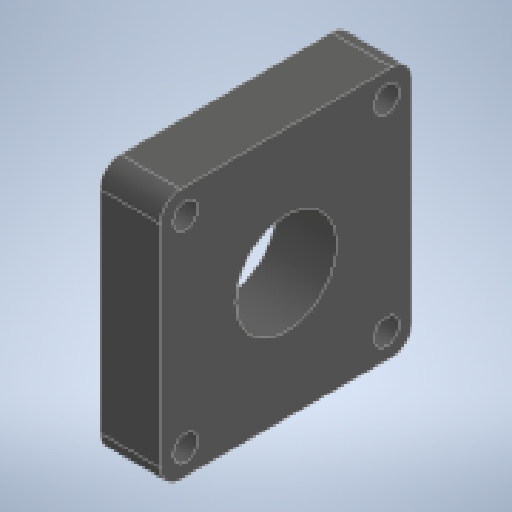
# Autodesk Inventor part: 25mmx25mmx6mm_fan
Saved by Autodesk Inventor 2024.1 (Build 281209000, 209)
## iProperties
Created: 2023-10-17
Part Number: 25mmx25mmx6mm_fan
Material: Generic
Document SubType Name: Modeling
Designer: l1534
Density: 1 g/cm^3
Appearance: Generic
Author: l1534
Autodesk Inventor part; units mm, degrees
ref_plane "YZ Plane" through (0, 0, 0) normal (1, 0, 0) x (0, 1, 0)
ref_plane "XZ Plane" through (0, 0, 0) normal (0, 1, 0) x (-1, 0, 0)
ref_plane "XY Plane" through (0, 0, 0) normal (0, 0, 1) x (1, 0, 0)
sketch "Sketch1" plane through (0, 0, 0) normal (1, 0, 0) x (0, 1, 0)
  line L0 (12.7439, 15.061) -> (-12.2561, 15.061)
  line L1 (-12.2561, 15.061) -> (-12.2561, -9.939)
  line L2 (-12.2561, -9.939) -> (12.7439, -9.939)
  line L3 (12.7439, -9.939) -> (12.7439, 15.061)
  point P0 (0, 0)
  dimension "d0" = 25
  dimension "d1" = 25
  constraints: 8 end point, 2 parallel, 1 horizontal, 1 perpendicular
  measures "d0" distance of L0.start L0.end
  measures "d1" distance of L0.end L1.end
extrude "Extrusion1" add sketch "Sketch1" along normal blind 6
fillet "Fillet1" radius 2 4 edges at (3, -12.2561, 15.061) (3, 12.7439, 15.061) (3, -12.2561, -9.939) (3, 12.7439, -9.939)
sketch "Sketch2" plane through (0, 0, 0) normal (-1, 0, 0) x (0, 0, 1)
  circle A0 centre (12.561, 10.2439) radius 1.25
  circle A1 centre (12.561, -9.7561) radius 1.25
  circle A2 centre (-7.439, -9.7561) radius 1.25
  circle A3 centre (-7.439, 10.2439) radius 1.25
  line L0 (15.061, 10.7439) -> (15.061, -10.2561) projected
  line L1 (-7.939, 12.7439) -> (13.061, 12.7439) projected
  line L2 (13.061, -12.2561) -> (-7.939, -12.2561) projected
  line L3 (-9.939, -10.2561) -> (-9.939, 10.7439) projected
  point P0 (0, 0)
  dimension "d5" = 2.5
  dimension "d6" = 2.5
  dimension "d7" = 2.5
  dimension "d8" = 2.5
  dimension "d9" = 2.5
  dimension "d10" = 2.5
  dimension "d11" = 2.5
  dimension "d12" = 2.5
  dimension "d13" = 2.5
  dimension "d14" = 2.5
  dimension "d15" = 2.5
  dimension "d16" = 2.5
  constraints: 4 centre point
  measures "d5" diameter of A1
  measures "d6" diameter of A2
  measures "d7" diameter of A3
  measures "d8" diameter of A0
  measures "d9" distance from line of L0 A0.centre
  measures "d10" distance from line of L1 A0.centre
  measures "d11" distance from line of L2 A1.centre
  measures "d12" distance from line of L0 A1.centre
  measures "d13" distance from line of L2 A2.centre
  measures "d14" distance from line of L3 A2.centre
  measures "d15" distance from line of L3 A3.centre
  measures "d16" distance from line of L1 A3.centre
extrude "Extrusion2" cut sketch "Sketch2" against normal through all
sketch "Sketch3" plane through (0, 0, 0) normal (-1, 0, 0) x (0, 0, 1)
  circle A0 centre (2.561, 0.2439) radius 5
  line L0 (13.061, -12.2561) -> (-7.939, -12.2561) projected
  line L1 (15.061, 10.7439) -> (15.061, -10.2561) projected
  point P0 (0, 0)
  dimension "d19" = 10
  dimension "d20" = 12.5
  dimension "d21" = 12.5
  constraints: 1 centre point
  measures "d19" diameter of A0
  measures "d20" distance from line of L0 A0.centre
  measures "d21" distance from line of L1 A0.centre
extrude "Extrusion3" cut sketch "Sketch3" against normal blind 10
body "Solid1"
